Autodesk Fusion 360 part; units mm, degrees
(part 3 of 7)
  line L316 (-32.3491, 29.3042) -> (-32.304, 29.3816)
  spline S628 degree 2 poles (-32.304, 29.3816) (-33.5803, 30.3455) (-33.8371, 31.9456) knots 0 0 0 1 1 1
  spline S629 degree 2 poles (-33.8371, 31.9456) (-33.0539, 30.266) (-32.1923, 29.5954) knots 0 0 0 1 1 1
  line L317 (-32.1923, 29.5954) -> (-32.0902, 29.6502)
  spline S630 degree 2 poles (-32.0902, 29.6502) (-33.142, 30.468) (-33.445, 31.9123) knots 0 0 0 1 1 1
  spline S631 degree 2 poles (-33.445, 31.9123) (-32.5168, 30.1435) (-31.7765, 29.6621) knots 0 0 0 1 1 1
  line L318 (-31.7765, 29.6621) -> (-31.71, 29.7845)
  spline S632 degree 2 poles (-31.71, 29.7845) (-32.8852, 30.77) (-33.0303, 31.7339) knots 0 0 0 1 1 1
  spline S633 degree 2 poles (-33.0303, 31.7339) (-32.3137, 30.4562) (-31.6649, 30.0091) knots 0 0 0 1 1 1
  line L319 (-31.6649, 30.0091) -> (-31.609, 30.0865)
  spline S634 degree 2 poles (-31.609, 30.0865) (-32.2364, 30.6238) (-32.5265, 31.4652) knots 0 0 0 1 1 1
  spline S635 degree 2 poles (-32.5265, 31.4652) (-32.1118, 30.7581) (-31.4403, 30.2326) knots 0 0 0 1 1 1
  line L320 (-31.4403, 30.2326) -> (-31.3844, 30.3337)
  spline S636 degree 2 poles (-31.3844, 30.3337) (-31.8099, 30.871) (-32.1118, 31.4416) knots 0 0 0 1 1 1
  spline S637 degree 2 poles (-32.1118, 31.4416) (-31.5691, 30.7581) (-31.2878, 30.5905) knots 0 0 0 1 1 1
  line L321 (-31.2878, 30.5905) -> (-31.1878, 30.7248)
  spline S638 degree 2 poles (-31.1878, 30.7248) (-31.406, 31.0268) (-31.5284, 31.3868) knots 0 0 0 1 1 1
  spline S639 degree 3 poles (-31.5284, 31.3868) (-31.6519, 31.7446) (-31.0868, 30.9387) (-30.9419, 30.8258) knots 0 0 0 0 1 1 1 1
  line L322 (-30.9419, 30.8258) -> (-30.9074, 30.872)
  spline S640 degree 2 poles (-30.9074, 30.872) (-31.1374, 31.1848) (-31.3049, 31.5093) knots 0 0 0 1 1 1
  spline S641 degree 3 poles (-31.3049, 31.5093) (-31.4725, 31.8327) (-31.2662, 31.6705) (-30.7625, 31.1117) knots 0 0 0 0 1 1 1 1
  line L323 (-30.7625, 31.1117) -> (-30.7066, 31.2234)
  spline S642 degree 2 poles (-30.7066, 31.2234) (-31.2545, 32.2486) (-30.6282, 31.5308) knots 0 0 0 1 1 1
  spline S643 degree 2 poles (-30.6282, 31.5308) (-30.4433, 31.7113) (-30.801, 32.081) knots 0 0 0 1 1 1
  spline S644 degree 3 poles (-30.801, 32.081) (-31.1588, 32.4506) (-30.5207, 32.081) (-30.3198, 31.7349) knots 0 0 0 0 1 1 1 1
  spline S645 degree 3 poles (-30.3198, 31.7349) (-30.1179, 31.3878) (-30.2628, 32.0143) (-30.6454, 32.4377) knots 0 0 0 0 1 1 1 1
  spline S646 degree 3 poles (-30.6454, 32.4377) (-31.0256, 32.8633) (-30.5217, 32.6182) (-30.4541, 32.528) knots 0 0 0 0 1 1 1 1
  spline S647 degree 2 poles (-30.4541, 32.528) (-30.3865, 32.4377) (-30.2199, 32.2368) knots 0 0 0 1 1 1
  spline S648 degree 2 poles (-30.2199, 32.2368) (-30.3231, 32.6859) (-30.6689, 33.0653) knots 0 0 0 1 1 1
  spline S649 degree 3 poles (-30.6689, 33.0653) (-31.017, 33.4457) (-30.5809, 33.1771) (-30.4917, 33.0653) knots 0 0 0 0 1 1 1 1
  spline S650 degree 3 poles (-30.4917, 33.0653) (-30.4015, 32.9535) (-30.2896, 32.874) (-30.1318, 32.6311) knots 0 0 0 0 1 1 1 1
  spline S651 degree 2 poles (-30.1318, 32.6311) (-30.165, 33.0213) (-30.5357, 33.3682) knots 0 0 0 1 1 1
  spline S652 degree 3 poles (-30.5357, 33.3682) (-30.9053, 33.7143) (-30.3574, 33.5467) (-30.0888, 33.1437) knots 0 0 0 0 1 1 1 1
  spline S653 degree 2 poles (-30.0888, 33.1437) (-29.9546, 33.2447) (-30.4917, 33.9497) knots 0 0 0 1 1 1
  spline S654 degree 2 poles (-30.4917, 33.9497) (-31.0289, 34.6546) (-29.9975, 33.58) knots 0 0 0 1 1 1
  spline S655 degree 2 poles (-29.9975, 33.58) (-29.8471, 33.6326) (-30.2887, 34.1303) knots 0 0 0 1 1 1
  spline S656 degree 2 poles (-30.2887, 34.1303) (-30.6474, 34.5331) (-29.9642, 34.04) knots 0 0 0 1 1 1
  spline S657 degree 2 poles (-29.9642, 34.04) (-29.8524, 34.1527) (-30.1102, 34.5203) knots 0 0 0 1 1 1
  spline S658 degree 3 poles (-30.1102, 34.5203) (-30.3563, 34.8727) (-30.0094, 34.6546) (-29.9535, 34.5868) knots 0 0 0 0 1 1 1 1
  spline S659 degree 3 poles (-29.9535, 34.5868) (-29.8954, 34.5203) (-29.8954, 34.9222) (-30.0877, 35.0801) knots 0 0 0 0 1 1 1 1
  spline S660 degree 3 poles (-30.0877, 35.0801) (-30.2779, 35.237) (-30.0094, 35.2478) (-29.9308, 35.1704) knots 0 0 0 0 1 1 1 1
  spline S661 degree 3 poles (-29.9308, 35.1704) (-29.8524, 35.0931) (-29.8524, 35.3048) (-30.0426, 35.5272) knots 0 0 0 0 1 1 1 1
  spline S662 degree 3 poles (-30.0426, 35.5272) (-30.2328, 35.7517) (-29.8858, 35.5842) (-29.8513, 35.5518) knots 0 0 0 0 1 1 1 1
  spline S663 degree 3 poles (-29.8513, 35.5518) (-29.8192, 35.5164) (-29.774, 35.6508) (-29.9083, 35.8206) knots 0 0 0 0 1 1 1 1
  spline S664 degree 3 poles (-29.9083, 35.8206) (-30.0426, 35.9881) (-29.8062, 35.9549) (-29.7611, 35.8754) knots 0 0 0 0 1 1 1 1
  spline S665 degree 3 poles (-29.7611, 35.8754) (-29.717, 35.7959) (-29.6462, 35.9549) (-29.7278, 36.0429) knots 0 0 0 0 1 1 1 1
  spline S666 degree 3 poles (-29.7278, 36.0429) (-29.918, 36.2408) (-29.5345, 36.0623) (-29.4775, 36.158) knots 0 0 0 0 1 1 1 1
  spline S667 degree 3 poles (-29.4775, 36.158) (-29.6622, 36.532) (-29.8342, 36.576) (-30.1265, 36.6222) knots 0 0 0 0 1 1 1 1
  spline S668 degree 3 poles (-30.1265, 36.6222) (-30.4036, 36.6641) (-30.8591, 36.4965) (-31.1136, 36.3847) knots 0 0 0 0 1 1 1 1
  spline S669 degree 2 poles (-31.1136, 36.3847) (-31.161, 36.2397) (-31.0933, 36.0526) knots 0 0 0 1 1 1
  spline S670 degree 3 poles (-31.0933, 36.0526) (-30.9364, 35.6282) (-31.205, 35.9872) (-31.1836, 35.8968) knots 0 0 0 0 1 1 1 1
  spline S671 degree 3 poles (-31.1836, 35.8968) (-31.161, 35.8065) (-31.1266, 35.5509) (-31.2276, 35.683) knots 0 0 0 0 1 1 1 1
  spline S672 degree 2 poles (-31.2276, 35.683) (-31.3285, 35.8195) (-31.4628, 35.9291) knots 0 0 0 1 1 1
  line L324 (-31.4628, 35.9291) -> (-31.4575, 35.9485)
  spline S673 degree 3 poles (-31.4575, 35.9485) (-31.4673, 35.9688) (-31.4706, 35.9917) (-31.4672, 36.014) knots 0 0 0 0 1 1 1 1
  spline S674 degree 3 poles (-31.4672, 36.014) (-31.4274, 36.3073) (-31.4704, 36.4986) (-31.5918, 36.5868) knots 0 0 0 0 1 1 1 1
  spline S675 degree 3 poles (-31.5918, 36.5868) (-31.7142, 36.6749) (-31.9141, 36.6577) (-32.0902, 36.6115) knots 0 0 0 0 1 1 1 1
  spline S676 degree 3 poles (-32.0902, 36.6115) (-32.2696, 36.4061) (-32.4147, 35.6883) (-32.4147, 35.5261) knots 0 0 0 0 1 1 1 1
  spline S677 degree 3 poles (-32.4147, 35.5261) (-32.4147, 35.3606) (-32.2685, 35.0017) (-32.2685, 34.8232) knots 0 0 0 0 1 1 1 1
  spline S678 degree 3 poles (-32.2685, 34.8232) (-32.2685, 34.6449) (-32.3706, 34.6449) (-32.4028, 34.733) knots 0 0 0 0 1 1 1 1
  spline S679 degree 3 poles (-32.4028, 34.733) (-32.4362, 34.8234) (-32.5146, 35.1135) (-32.5941, 35.2478) knots 0 0 0 0 1 1 1 1
  spline S680 degree 3 poles (-32.5941, 35.2478) (-32.6714, 35.3821) (-32.7606, 35.8206) (-32.7606, 35.9634) knots 0 0 0 0 1 1 1 1
  spline S681 degree 3 poles (-32.7606, 35.9634) (-32.7606, 36.1107) (-32.6714, 36.2784) (-32.6714, 36.3793) knots 0 0 0 0 1 1 1 1
  spline S682 degree 3 poles (-32.6714, 36.3793) (-32.6714, 36.4761) (-32.6714, 36.606) (-32.7843, 36.6652) knots 0 0 0 0 1 1 1 1
  spline S683 degree 3 poles (-32.7843, 36.6652) (-32.8667, 36.6822) (-32.952, 36.68) (-33.0335, 36.6588) knots 0 0 0 0 1 1 1 1
  spline S684 degree 3 poles (-33.0335, 36.6588) (-33.0549, 36.6507) (-33.0773, 36.6457) (-33.1001, 36.6436) knots 0 0 0 0 1 1 1 1
  spline S685 degree 3 poles (-33.1001, 36.6436) (-33.0722, 36.5954) (-33.0109, 36.534) (-32.9733, 36.3997) knots 0 0 0 0 1 1 1 1
  spline S686 degree 2 poles (-32.9733, 36.3997) (-32.9175, 36.1977) (-33.0969, 36.2106) knots 0 0 0 1 1 1
  spline S687 degree 2 poles (-33.0969, 36.2106) (-33.0292, 36.0429) (-33.2752, 36.1096) knots 0 0 0 1 1 1
  spline S688 degree 2 poles (-33.2752, 36.1096) (-33.1979, 35.8979) (-33.4772, 36.0323) knots 0 0 0 1 1 1
  spline S689 degree 2 poles (-33.4772, 36.0323) (-33.3998, 35.7195) (-33.7006, 35.9549) knots 0 0 0 1 1 1
  spline S690 degree 2 poles (-33.7006, 35.9549) (-33.4879, 35.4831) (-33.8242, 35.7195) knots 0 0 0 1 1 1
  spline S691 degree 2 poles (-33.8242, 35.7195) (-33.735, 35.3251) (-33.9026, 35.3918) knots 0 0 0 1 1 1
  spline S692 degree 2 poles (-33.9026, 35.3918) (-33.8349, 35.1693) (-34.0251, 35.2263) knots 0 0 0 1 1 1
  spline S693 degree 3 poles (-34.0251, 35.2263) (-34.0025, 35.1576) (-34.0025, 34.9447) (-34.1819, 35.0233) knots 0 0 0 0 1 1 1 1
  spline S694 degree 2 poles (-34.1819, 35.0233) (-34.3613, 35.1027) (-34.3388, 35.2811) knots 0 0 0 1 1 1
  spline S695 degree 3 poles (-34.3388, 35.2811) (-34.1819, 35.2918) (-34.2378, 35.4175) (-34.2496, 35.5604) knots 0 0 0 0 1 1 1 1
  spline S696 degree 3 poles (-34.2496, 35.5604) (-34.2604, 35.7077) (-34.3388, 35.8206) (-34.2937, 35.7851) knots 0 0 0 0 1 1 1 1
  spline S697 degree 3 poles (-34.2937, 35.7851) (-34.1046, 35.6443) (-34.2152, 35.9881) (-34.2937, 36.0763) knots 0 0 0 0 1 1 1 1
  spline S698 degree 3 poles (-34.2937, 36.0763) (-34.3721, 36.1666) (-34.3613, 36.3321) (-34.3162, 36.3009) knots 0 0 0 0 1 1 1 1
  spline S699 degree 3 poles (-34.3162, 36.3009) (-34.0874, 36.129) (-34.1819, 36.3665) (-34.2937, 36.6007) knots 0 0 0 0 1 1 1 1
  spline S700 degree 2 poles (-34.2937, 36.6007) (-34.4065, 36.8382) (-34.1927, 36.7244) knots 0 0 0 1 1 1
  spline S701 degree 2 poles (-34.1927, 36.7244) (-34.0702, 36.5791) (-34.1712, 36.8146) knots 0 0 0 1 1 1
  spline S702 degree 3 poles (-34.1712, 36.8146) (-34.2851, 37.079) (-34.1336, 37.079) (-34.0852, 37.0746) knots 0 0 0 0 1 1 1 1
  spline S703 degree 3 poles (-34.0852, 37.0746) (-34.0928, 37.2304) (-34.1346, 37.4508) (-34.3022, 37.4948) knots 0 0 0 0 1 1 1 1
  spline S704 degree 3 poles (-34.3022, 37.4948) (-34.5203, 37.5571) (-35.166, 37.2067) (-35.5925, 36.9779) knots 0 0 0 0 1 1 1 1
  spline S705 degree 2 poles (-31.3082, 35.3262) (-31.2631, 35.5948) (-31.4425, 35.7861) knots 0 0 0 1 1 1
  spline S706 degree 3 poles (-31.4425, 35.7861) (-31.6219, 35.9773) (-31.5768, 35.7968) (-31.5435, 35.7088) knots 0 0 0 0 1 1 1 1
  spline S707 degree 3 poles (-31.5435, 35.7088) (-31.509, 35.6174) (-31.4425, 35.4389) (-31.3082, 35.3262) knots 0 0 0 0 1 1 1 1
  spline S708 degree 2 poles (-31.5317, 35.1919) (-31.5101, 35.5378) (-31.7003, 35.5067) knots 0 0 0 1 1 1
  spline S709 degree 3 poles (-31.7003, 35.5067) (-31.767, 35.4959) (-31.6327, 35.3047) (-31.5317, 35.1919) knots 0 0 0 0 1 1 1 1
  spline S710 degree 2 poles (-31.6433, 34.9016) (-31.6433, 35.1488) (-31.7776, 35.2144) knots 0 0 0 1 1 1
  spline S711 degree 3 poles (-31.7776, 35.2144) (-32.043, 35.3467) (-31.7111, 34.9586) (-31.6433, 34.9016) knots 0 0 0 0 1 1 1 1
  spline S712 degree 2 poles (-31.7776, 34.7104) (-31.8121, 34.9899) (-31.9345, 34.9458) knots 0 0 0 1 1 1
  spline S713 degree 3 poles (-31.9345, 34.9458) (-32.058, 34.9016) (-31.8335, 34.7341) (-31.7776, 34.7104) knots 0 0 0 0 1 1 1 1
  spline S714 degree 2 poles (-31.9689, 36.4191) (-31.7787, 36.4319) (-31.6884, 36.3857) knots 0 0 0 1 1 1
  spline S715 degree 2 poles (-31.6884, 36.3857) (-31.7454, 36.577) (-31.9689, 36.4191) knots 0 0 0 1 1 1
  spline S716 degree 2 poles (-31.7111, 36.2664) (-31.8572, 36.3922) (-31.9689, 36.3126) knots 0 0 0 1 1 1
  spline S717 degree 2 poles (-31.9689, 36.3126) (-32.0807, 36.2331) (-31.7111, 36.2664) knots 0 0 0 1 1 1
  spline S718 degree 2 poles (-31.7562, 36.1547) (-31.8572, 36.1107) (-31.9345, 36.1107) knots 0 0 0 1 1 1
  spline S719 degree 3 poles (-31.9345, 36.1107) (-32.0129, 36.1107) (-31.8678, 35.9978) (-31.7562, 36.1547) knots 0 0 0 0 1 1 1 1
  spline S720 degree 2 poles (-34.2292, 34.9791) (-34.3635, 34.9685) (-34.3635, 34.8781) knots 0 0 0 1 1 1
  spline S721 degree 2 poles (-34.3635, 34.8781) (-34.2958, 34.935) (-34.1948, 34.8448) knots 0 0 0 1 1 1
  spline S722 degree 2 poles (-34.1948, 34.8448) (-34.0949, 34.7545) (-34.2292, 34.9791) knots 0 0 0 1 1 1
  spline S723 degree 2 poles (-31.5209, 31.9004) (-31.6424, 32.0477) (-31.6552, 32.1272) knots 0 0 0 1 1 1
  spline S724 degree 3 poles (-31.6552, 32.1272) (-31.6659, 32.2035) (-31.5209, 32.0939) (-31.5209, 31.9004) knots 0 0 0 0 1 1 1 1
  spline S725 degree 2 poles (-31.6499, 31.4523) (-31.7723, 31.5985) (-31.7841, 31.6759) knots 0 0 0 1 1 1
  spline S726 degree 3 poles (-31.7841, 31.6759) (-31.7949, 31.7543) (-31.6499, 31.6447) (-31.6499, 31.4523) knots 0 0 0 0 1 1 1 1
  spline S727 degree 2 poles (-31.0676, 31.9445) (-31.1911, 32.0917) (-31.2019, 32.1691) knots 0 0 0 1 1 1
  spline S728 degree 3 poles (-31.2019, 32.1691) (-31.2147, 32.2475) (-31.0676, 32.1379) (-31.0676, 31.9445) knots 0 0 0 0 1 1 1 1
  spline S729 degree 2 poles (-31.0117, 32.3496) (-31.1352, 32.4968) (-31.146, 32.5721) knots 0 0 0 1 1 1
  spline S730 degree 3 poles (-31.146, 32.5721) (-31.1578, 32.6515) (-31.0117, 32.5409) (-31.0117, 32.3496) knots 0 0 0 0 1 1 1 1
  spline S731 degree 2 poles (-30.8946, 32.7655) (-30.9505, 32.8536) (-30.9945, 32.8998) knots 0 0 0 1 1 1
  spline S732 degree 3 poles (-30.9945, 32.8998) (-31.0396, 32.9438) (-30.827, 32.9438) (-30.8946, 32.7655) knots 0 0 0 0 1 1 1 1
  spline S733 degree 2 poles (-31.3641, 32.283) (-31.4209, 32.3711) (-31.465, 32.4173) knots 0 0 0 1 1 1
  spline S734 degree 3 poles (-31.465, 32.4173) (-31.5092, 32.4614) (-31.2963, 32.4614) (-31.3641, 32.283) knots 0 0 0 0 1 1 1 1
  spline S735 degree 2 poles (-32.2031, 31.6995) (-32.2601, 31.7919) (-32.3041, 31.8338) knots 0 0 0 1 1 1
  spline S736 degree 3 poles (-32.3041, 31.8338) (-32.3493, 31.88) (-32.1364, 31.88) (-32.2031, 31.6995) knots 0 0 0 0 1 1 1 1
  spline S737 degree 2 poles (-32.606, 31.6909) (-32.663, 31.779) (-32.707, 31.8252) knots 0 0 0 1 1 1
  spline S738 degree 3 poles (-32.707, 31.8252) (-32.7521, 31.8693) (-32.5383, 31.8693) (-32.606, 31.6909) knots 0 0 0 0 1 1 1 1
  spline S739 degree 2 poles (-30.4014, 34.3977) (-30.4574, 34.486) (-30.5025, 34.5322) knots 0 0 0 1 1 1
  spline S740 degree 3 poles (-30.5025, 34.5322) (-30.5476, 34.5762) (-30.3349, 34.5762) (-30.4014, 34.3977) knots 0 0 0 0 1 1 1 1
  spline S741 degree 2 poles (-30.2458, 34.7803) (-30.3006, 34.8685) (-30.3466, 34.9147) knots 0 0 0 1 1 1
  spline S742 degree 3 poles (-30.3466, 34.9147) (-30.3897, 34.9588) (-30.178, 34.9588) (-30.2458, 34.7803) knots 0 0 0 0 1 1 1 1
  line L325 (-32.4609, 32.182) -> (-32.405, 32.1379)
  line L326 (-32.405, 32.1379) -> (-32.3944, 32.2615)
  line L327 (-32.3944, 32.2615) -> (-32.4609, 32.2723)
  line L328 (-32.4609, 32.2723) -> (-32.4609, 32.182)
  line L329 (-31.8368, 32.3625) -> (-31.7809, 32.3163)
  line L330 (-31.7809, 32.3163) -> (-31.769, 32.4399)
  line L331 (-31.769, 32.4399) -> (-31.8368, 32.4528)
  line L332 (-31.8368, 32.4528) -> (-31.8368, 32.3625)
  line L333 (-30.972, 34.0163) -> (-30.9172, 33.9744)
  line L334 (-30.9172, 33.9744) -> (-30.9053, 34.0959)
  line L335 (-30.9053, 34.0959) -> (-30.972, 34.1087)
  line L336 (-30.972, 34.1087) -> (-30.972, 34.0163)
  line L337 (-30.7152, 33.7605) -> (-30.6583, 33.7144)
  line L338 (-30.6583, 33.7144) -> (-30.6486, 33.8401)
  line L339 (-30.6486, 33.8401) -> (-30.7152, 33.8487)
  line L340 (-30.7152, 33.8487) -> (-30.7152, 33.7605)
  spline S743 degree 3 poles (-43.5424, 38.6843) (-43.5791, 38.6514) (-43.6163, 38.6192) (-43.6541, 38.5875) knots 0 0 0 0 1 1 1 1
  line L341 (-43.6541, 38.5875) -> (-43.6541, 33.162)
  spline S744 degree 3 poles (-43.6541, 33.162) (-43.6187, 33.25) (-43.5811, 33.3381) (-43.5424, 33.4285) knots 0 0 0 0 1 1 1 1
  line L342 (-43.5424, 33.4285) -> (-43.5424, 38.6843)
  line L343 (-44.4846, 37.8107) -> (-44.5974, 37.6956)
  line L344 (-44.5974, 37.6956) -> (-44.5974, 32.4302)
  line L345 (-44.5974, 32.4302) -> (-44.4846, 32.4011)
  line L346 (-44.4846, 32.4011) -> (-44.4846, 37.8107)
  line L347 (-43.2276, 38.9401) -> (-43.3404, 38.8477)
  line L348 (-43.3404, 38.8477) -> (-43.3404, 33.84)
  spline S745 degree 3 poles (-43.3404, 33.84) (-43.3039, 33.9067) (-43.2663, 33.9764) (-43.2276, 34.0431) knots 0 0 0 0 1 1 1 1
  line L349 (-43.2276, 34.0431) -> (-43.2276, 38.9401)
  spline S746 degree 3 poles (-44.1698, 38.1213) (-44.2084, 38.0858) (-44.246, 38.0493) (-44.2826, 38.0117) knots 0 0 0 0 1 1 1 1
  line L350 (-44.2826, 38.0117) -> (-44.2826, 32.341)
  line L351 (-44.2826, 32.341) -> (-44.1698, 32.3076)
  line L352 (-44.1698, 32.3076) -> (-44.1698, 38.1213)
  spline S747 degree 3 poles (-45.4267, 36.7317) (-45.4654, 36.6813) (-45.503, 36.6329) (-45.5395, 36.5824) knots 0 0 0 0 1 1 1 1
  line L353 (-45.5395, 36.5824) -> (-45.5395, 32.6999)
  line L354 (-45.5395, 32.6999) -> (-45.4267, 32.6687)
  line L355 (-45.4267, 32.6687) -> (-45.4267, 36.7317)
  spline S748 degree 3 poles (-45.7404, 36.3062) (-45.7785, 36.2522) (-45.8161, 36.1977) (-45.8532, 36.1429) knots 0 0 0 0 1 1 1 1
  line L356 (-45.8532, 36.1429) -> (-45.8532, 32.7913)
  line L357 (-45.8532, 32.7913) -> (-45.7404, 32.76)
  line L358 (-45.7404, 32.76) -> (-45.7404, 36.3062)
  spline S749 degree 3 poles (-45.1119, 37.1208) (-45.1507, 37.0762) (-45.1883, 37.0307) (-45.2247, 36.9843) knots 0 0 0 0 1 1 1 1
  line L359 (-45.2247, 36.9843) -> (-45.2247, 32.6107)
  line L360 (-45.2247, 32.6107) -> (-45.1119, 32.5795)
  line L361 (-45.1119, 32.5795) -> (-45.1119, 37.1208)
  line L362 (-44.7993, 37.4797) -> (-44.9111, 37.3529)
  line L363 (-44.9111, 37.3529) -> (-44.9111, 32.5193)
  line L364 (-44.9111, 32.5193) -> (-44.7993, 32.4882)
  line L365 (-44.7993, 32.4882) -> (-44.7993, 37.4797)
  spline S750 degree 3 poles (-40.7137, 40.525) (-40.7518, 40.5077) (-40.7894, 40.4894) (-40.8265, 40.4702) knots 0 0 0 0 1 1 1 1
  line L366 (-40.8265, 40.4702) -> (-40.8265, 36.9381)
  line L367 (-40.8265, 36.9381) -> (-40.7137, 37.0198)
  line L368 (-40.7137, 37.0198) -> (-40.7137, 40.525)
  line L369 (-41.6559, 40.0146) -> (-41.7687, 39.9481)
  line L370 (-41.7687, 39.9481) -> (-41.7687, 36.057)
  line L371 (-41.7687, 36.057) -> (-41.6559, 36.1869)
  line L372 (-41.6559, 36.1869) -> (-41.6559, 40.0146)
  line L373 (-40.0853, 40.8206) -> (-40.1981, 40.77)
  line L374 (-40.1981, 40.77) -> (-40.1981, 37.3324)
  spline S751 degree 3 poles (-40.1981, 37.3324) (-40.1594, 37.3518) (-40.1218, 37.3722) (-40.0853, 37.3894) knots 0 0 0 0 1 1 1 1
  line L375 (-40.0853, 37.3894) -> (-40.0853, 40.8206)
  line L376 (-40.399, 40.6776) -> (-40.5118, 40.6229)
  line L377 (-40.5118, 40.6229) -> (-40.5118, 37.1497)
  spline S752 degree 3 poles (-40.5118, 37.1497) (-40.4742, 37.1724) (-40.4366, 37.1981) (-40.399, 37.2186) knots 0 0 0 0 1 1 1 1
  line L378 (-40.399, 37.2186) -> (-40.399, 40.6776)
  spline S753 degree 3 poles (-42.5991, 39.4064) (-42.6376, 39.3816) (-42.6748, 39.355) (-42.7109, 39.3269) knots 0 0 0 0 1 1 1 1
  line L379 (-42.7109, 39.3269) -> (-42.7109, 34.849)
  line L380 (-42.7109, 34.849) -> (-42.5991, 35.0059)
  line L381 (-42.5991, 35.0059) -> (-42.5991, 39.4064)
  spline S754 degree 3 poles (-42.9128, 39.1797) (-42.9509, 39.1525) (-42.9886, 39.1245) (-43.0256, 39.0958) knots 0 0 0 0 1 1 1 1
  line L382 (-43.0256, 39.0958) -> (-43.0256, 34.3817)
  line L383 (-43.0256, 34.3817) -> (-42.9128, 34.5558)
  line L384 (-42.9128, 34.5558) -> (-42.9128, 39.1797)
  line L385 (-41.9707, 39.8233) -> (-42.0835, 39.7524)
  line L386 (-42.0835, 39.7524) -> (-42.0835, 35.6764)
  line L387 (-42.0835, 35.6764) -> (-41.9707, 35.8151)
  line L388 (-41.9707, 35.8151) -> (-41.9707, 39.8233)
  spline S755 degree 3 poles (-42.2844, 39.6223) (-42.3225, 39.5973) (-42.3601, 39.5716) (-42.3972, 39.545) knots 0 0 0 0 1 1 1 1
  line L389 (-42.3972, 39.545) -> (-42.3972, 35.2778)
  line L390 (-42.3972, 35.2778) -> (-42.2844, 35.4229)
  line L391 (-42.2844, 35.4229) -> (-42.2844, 39.6223)
  line L392 (-41.0274, 40.365) -> (-41.1402, 40.3038)
  line L393 (-41.1402, 40.3038) -> (-41.1402, 36.6899)
  spline S756 degree 3 poles (-41.1402, 36.6899) (-41.1026, 36.7211) (-41.065, 36.7532) (-41.0274, 36.7823) knots 0 0 0 0 1 1 1 1
  line L394 (-41.0274, 36.7823) -> (-41.0274, 40.365)
  spline S757 degree 3 poles (-29.4024, 41.7502) (-29.44, 41.7608) (-29.4775, 41.7694) (-29.5151, 41.777) knots 0 0 0 0 1 1 1 1
  line L395 (-29.5151, 41.777) -> (-29.5151, 36.6179)
  spline S758 degree 3 poles (-29.5151, 36.6179) (-29.473, 36.5795) (-29.4352, 36.5365) (-29.4024, 36.49) knots 0 0 0 0 1 1 1 1
  line L396 (-29.4024, 36.49) -> (-29.4024, 41.7502)
  spline S759 degree 3 poles (-30.0309, 41.8866) (-30.0684, 41.8952) (-30.106, 41.9016) (-30.1436, 41.908) knots 0 0 0 0 1 1 1 1
  line L397 (-30.1436, 41.908) -> (-30.1436, 36.8607)
  line L398 (-30.1436, 36.8607) -> (-30.0932, 36.8543)
  line L399 (-30.0932, 36.8543) -> (-30.0298, 36.8435)
  line L400 (-30.0298, 36.8435) -> (-30.0298, 41.8866)
  line L401 (-30.0298, 41.8866) -> (-30.0309, 41.8866)
  spline S760 degree 3 poles (-29.0887, 41.6727) (-29.1263, 41.6835) (-29.1627, 41.6921) (-29.2003, 41.6996) knots 0 0 0 0 1 1 1 1
  line L402 (-29.2003, 41.6996) -> (-29.2003, 36.1171)
  spline S761 degree 3 poles (-29.2003, 36.1171) (-29.1616, 36.0242) (-29.1254, 35.9303) (-29.0918, 35.8356) knots 0 0 0 0 1 1 1 1
  line L403 (-29.0918, 35.8356) -> (-29.0876, 35.8206)
  line L404 (-29.0876, 35.8206) -> (-29.0887, 41.6727)
  line L405 (-33.8006, 42.2036) -> (-33.9144, 42.1993)
  line L406 (-33.9144, 42.1993) -> (-33.9144, 37.4033)
  spline S762 degree 3 poles (-33.9144, 37.4033) (-33.8667, 37.2679) (-33.8449, 37.1246) (-33.85, 36.9811) knots 0 0 0 0 1 1 1 1
  line L407 (-33.85, 36.9811) -> (-33.8006, 36.9639)
  line L408 (-33.8006, 36.9639) -> (-33.8006, 42.2036)
  line L409 (-35.7988, 42.0381) -> (-35.7988, 37.1336)
  line L410 (-35.7988, 37.1336) -> (-35.7042, 37.1842)
  line L411 (-35.7042, 37.1842) -> (-35.686, 37.1948)
  line L412 (-35.686, 37.1948) -> (-35.686, 42.0531)
  line L413 (-35.686, 42.0531) -> (-35.7988, 42.0381)
  spline S763 degree 3 poles (-46.0552, 35.8356) (-46.0936, 35.7751) (-46.1312, 35.7142) (-46.168, 35.6529) knots 0 0 0 0 1 1 1 1
  line L414 (-46.168, 35.6529) -> (-46.168, 32.8804)
  line L415 (-46.168, 32.8804) -> (-46.0552, 32.847)
  line L416 (-46.0552, 32.847) -> (-46.0552, 35.8356)
  line L417 (-27.9435, 38.2577) -> (-27.9435, 35.2756)
  spline S764 degree 3 poles (-27.9435, 35.2756) (-27.9274, 35.2775) (-27.9112, 35.2781) (-27.8951, 35.2778) knots 0 0 0 0 1 1 1 1
  spline S765 degree 3 poles (-27.8951, 35.2778) (-27.8746, 35.2778) (-27.8553, 35.28) (-27.8306, 35.2864) knots 0 0 0 0 1 1 1 1
  line L418 (-27.8306, 35.2864) -> (-27.8306, 38.1706)
  spline S766 degree 3 poles (-27.8306, 38.1706) (-27.8715, 38.1953) (-27.9093, 38.2245) (-27.9435, 38.2577) knots 0 0 0 0 1 1 1 1
  spline S767 degree 3 poles (-28.1809, 38.8186) (-28.1809, 38.9197) (-28.167, 39.0055) (-28.1443, 39.0786) knots 0 0 0 0 1 1 1 1
  line L419 (-28.1443, 39.0786) -> (-28.1443, 41.3976)
  line L420 (-28.1443, 41.3976) -> (-28.2581, 41.433)
  line L421 (-28.2581, 41.433) -> (-28.2581, 35.2692)
  spline S768 degree 3 poles (-28.2581, 35.2692) (-28.2196, 35.267) (-28.1819, 35.2692) (-28.1443, 35.2692) knots 0 0 0 0 1 1 1 1
  line L422 (-28.1443, 35.2692) -> (-28.1443, 38.5789)
  spline S769 degree 3 poles (-28.1443, 38.5789) (-28.1687, 38.6565) (-28.181, 38.7373) (-28.1809, 38.8186) knots 0 0 0 0 1 1 1 1
  line L423 (-27.315, 37.5613) -> (-27.315, 35.5927)
  spline S770 degree 3 poles (-27.315, 35.5927) (-27.2989, 35.606) (-27.2842, 35.6207) (-27.271, 35.6368) knots 0 0 0 0 1 1 1 1
  spline S771 degree 3 poles (-27.271, 35.6368) (-27.2483, 35.6561) (-27.2269, 35.6808) (-27.2032, 35.7077) knots 0 0 0 0 1 1 1 1
  line L424 (-27.2032, 35.7077) -> (-27.2032, 37.4055)
  line L425 (-27.2032, 37.4055) -> (-27.315, 37.5613)
  line L426 (-46.6837, 34.7029) -> (-46.7965, 34.4611)
  line L427 (-46.7965, 34.4611) -> (-46.7965, 33.0673)
  line L428 (-46.7965, 33.0673) -> (-46.718, 33.046)
  spline S772 degree 3 poles (-46.718, 33.046) (-46.7148, 33.0438) (-46.7116, 33.0416) (-46.7084, 33.0416) knots 0 0 0 0 1 1 1 1
  line L429 (-46.7084, 33.0416) -> (-46.6837, 33.033)
  line L430 (-46.6837, 33.033) -> (-46.6837, 34.7029)
  spline S773 degree 3 poles (-27.9435, 39.3978) (-27.9093, 39.4273) (-27.8718, 39.4526) (-27.8317, 39.4731) knots 0 0 0 0 1 1 1 1
  line L431 (-27.8317, 39.4731) -> (-27.8317, 41.2923)
  spline S774 degree 3 poles (-27.8317, 41.2923) (-27.8682, 41.3052) (-27.9059, 41.3192) (-27.9435, 41.33) knots 0 0 0 0 1 1 1 1
  line L432 (-27.9435, 41.33) -> (-27.9435, 39.3978)
  line L433 (-46.3689, 35.309) -> (-46.4817, 35.1037)
  line L434 (-46.4817, 35.1037) -> (-46.4817, 32.9738)
  line L435 (-46.4817, 32.9738) -> (-46.3689, 32.9427)
  line L436 (-46.3689, 32.9427) -> (-46.3689, 35.309)
  line L437 (-41.455, 40.1297) -> (-41.455, 36.3997)
  line L438 (-41.455, 36.3997) -> (-41.3422, 36.5093)
  line L439 (-41.3422, 36.5093) -> (-41.3422, 40.1952)
  spline S775 degree 3 poles (-41.3422, 40.1952) (-41.3798, 40.1737) (-41.4174, 40.1532) (-41.455, 40.1297) knots 0 0 0 0 1 1 1 1
  spline S776 degree 3 poles (-36.9429, 41.8318) (-36.9805, 41.8253) (-37.0181, 41.8167) (-37.0546, 41.8092) knots 0 0 0 0 1 1 1 1
  line L440 (-37.0546, 41.8092) -> (-37.0546, 37.1325)
  spline S777 degree 3 poles (-37.0546, 37.1325) (-37.0504, 37.1283) (-37.045, 37.1239) (-37.0407, 37.1175) knots 0 0 0 0 1 1 1 1
  spline S778 degree 3 poles (-37.0407, 37.1175) (-37.0262, 37.1021) (-37.0162, 37.083) (-37.0119, 37.0624) knots 0 0 0 0 1 1 1 1
  spline S779 degree 3 poles (-37.0119, 37.0624) (-37.0075, 37.0418) (-37.0089, 37.0203) (-37.016, 37.0004) knots 0 0 0 0 1 1 1 1
  spline S780 degree 3 poles (-37.016, 37.0004) (-37.0342, 36.9478) (-37.0482, 36.8554) (-37.0203, 36.8156) knots 0 0 0 0 1 1 1 1
  spline S781 degree 3 poles (-37.0203, 36.8156) (-37.0052, 36.7962) (-36.9719, 36.7909) (-36.9418, 36.7887) knots 0 0 0 0 1 1 1 1
  line L441 (-36.9418, 36.7887) -> (-36.9429, 41.8318)
  line L442 (-36.742, 41.8748) -> (-36.742, 36.7812)
  line L443 (-36.742, 36.7812) -> (-36.7367, 36.7812)
  spline S782 degree 3 poles (-36.7367, 36.7812) (-36.6948, 36.779) (-36.6625, 36.7768) (-36.6292, 36.779) knots 0 0 0 0 1 1 1 1
  line L444 (-36.6292, 36.779) -> (-36.6292, 41.8984)
  spline S783 degree 3 poles (-36.6292, 41.8984) (-36.6668, 41.8887) (-36.7044, 41.8823) (-36.742, 41.8748) knots 0 0 0 0 1 1 1 1
  line L445 (-43.9689, 38.3082) -> (-43.9689, 32.2507)
  line L446 (-43.9689, 32.2507) -> (-43.9356, 32.2399)
  spline S784 degree 3 poles (-43.9356, 32.2399) (-43.912, 32.3495) (-43.8851, 32.4559) (-43.855, 32.5613) knots 0 0 0 0 1 1 1 1
  line L447 (-43.855, 32.5613) -> (-43.855, 38.4125)
  spline S785 degree 3 poles (-43.855, 38.4125) (-43.8935, 38.3783) (-43.9314, 38.3435) (-43.9689, 38.3082) knots 0 0 0 0 1 1 1 1
  spline S786 degree 3 poles (-32.23, 42.1746) (-32.2665, 42.1768) (-32.3041, 42.1768) (-32.3416, 42.181) knots 0 0 0 0 1 1 1 1
  line L448 (-32.3416, 42.181) -> (-32.3416, 36.7812)
  spline S787 degree 3 poles (-32.3416, 36.7812) (-32.3083, 36.7962) (-32.2696, 36.8081) (-32.23, 36.821) knots 0 0 0 0 1 1 1 1
  line L449 (-32.23, 36.821) -> (-32.23, 42.1746)
  line L450 (-31.2878, 42.0865) -> (-31.3996, 42.0993)
  line L451 (-31.3996, 42.0993) -> (-31.3996, 36.7297)
  spline S788 degree 3 poles (-31.3996, 36.7297) (-31.3519, 36.6838) (-31.314, 36.629) (-31.2878, 36.5684) knots 0 0 0 0 1 1 1 1
  line L452 (-31.2878, 36.5684) -> (-31.2878, 42.0865)
  line L453 (-31.6004, 42.1198) -> (-31.7133, 42.1327)
  line L454 (-31.7133, 42.1327) -> (-31.7133, 36.8768)
  spline S789 degree 3 poles (-31.7133, 36.8768) (-31.675, 36.8704) (-31.6374, 36.8615) (-31.6004, 36.8499) knots 0 0 0 0 1 1 1 1
  line L455 (-31.6004, 36.8499) -> (-31.6004, 42.1198)
  line L456 (-30.9719, 42.0445) -> (-31.0848, 42.0617)
  line L457 (-31.0848, 42.0617) -> (-31.0848, 36.6533)
  spline S790 degree 3 poles (-31.0848, 36.6533) (-31.0504, 36.6683) (-31.0117, 36.6824) (-30.9719, 36.6973) knots 0 0 0 0 1 1 1 1
  line L458 (-30.9719, 36.6973) -> (-30.9719, 42.0445)
  line L459 (-30.6582, 42.0005) -> (-30.7711, 42.0155)
  line L460 (-30.7711, 42.0155) -> (-30.7711, 36.7662)
  line L461 (-30.7711, 36.7662) -> (-30.6582, 36.7973)
  line L462 (-30.6582, 36.7973) -> (-30.6582, 42.0005)
  spline S791 degree 3 poles (-31.9152, 42.1488) (-31.9517, 42.153) (-31.9904, 42.1552) (-32.0279, 42.1574) knots 0 0 0 0 1 1 1 1
  line L463 (-32.0279, 42.1574) -> (-32.0279, 36.8682)
  spline S792 degree 3 poles (-32.0279, 36.8682) (-31.9904, 36.8725) (-31.9528, 36.8789) (-31.9152, 36.8811) knots 0 0 0 0 1 1 1 1
  line L464 (-31.9152, 36.8811) -> (-31.9152, 42.1488)
  line L465 (-32.5437, 42.1885) -> (-32.6564, 42.195)
  line L466 (-32.6564, 42.195) -> (-32.6564, 36.8725)
  spline S793 degree 3 poles (-32.6564, 36.8725) (-32.6169, 36.8596) (-32.5789, 36.8419) (-32.5437, 36.8199) knots 0 0 0 0 1 1 1 1
  line L467 (-32.5437, 36.8199) -> (-32.5437, 42.1885)
  spline S794 degree 3 poles (-33.1721, 42.2078) (-33.2108, 42.21) (-33.2473, 42.21) (-33.286, 42.21) knots 0 0 0 0 1 1 1 1
  line L468 (-33.286, 42.21) -> (-33.286, 36.864)
  spline S795 degree 3 poles (-33.286, 36.864) (-33.2473, 36.864) (-33.2108, 36.8661) (-33.1732, 36.8704) knots 0 0 0 0 1 1 1 1
  line L469 (-33.1732, 36.8704) -> (-33.1721, 42.2078)
  line L470 (-32.8574, 36.9102) -> (-32.8574, 42.2014)
  spline S796 degree 3 poles (-32.8574, 42.2014) (-32.895, 42.2014) (-32.9325, 42.2036) (-32.9701, 42.2057) knots 0 0 0 0 1 1 1 1
  line L471 (-32.9701, 42.2057) -> (-32.9701, 36.9058)
  spline S797 degree 3 poles (-32.9701, 36.9058) (-32.9315, 36.9102) (-32.8939, 36.9122) (-32.8574, 36.9102) knots 0 0 0 0 1 1 1 1
  line L472 (-28.7739, 41.5889) -> (-28.8866, 41.6179)
  line L473 (-28.8866, 41.6179) -> (-28.8866, 35.4895)
  spline S798 degree 3 poles (-28.8866, 35.4895) (-28.8526, 35.4552) (-28.8148, 35.4249) (-28.7739, 35.3993) knots 0 0 0 0 1 1 1 1
  line L474 (-28.7739, 35.3993) -> (-28.7739, 41.5889)
  spline S799 degree 3 poles (-26.8884, 36.967) (-26.924, 37.0176) (-26.9615, 37.0724) (-27.0013, 37.1239) knots 0 0 0 0 1 1 1 1
  line L475 (-27.0013, 37.1239) -> (-27.0013, 35.9967)
  spline S800 degree 3 poles (-27.0013, 35.9967) (-26.9509, 36.0935) (-26.91, 36.202) (-26.8884, 36.3202) knots 0 0 0 0 1 1 1 1
  line L476 (-26.8884, 36.3202) -> (-26.8884, 36.967)
  line L477 (-27.5169, 37.8365) -> (-27.6298, 37.9857)
  line L478 (-27.6298, 37.9857) -> (-27.6298, 35.3659)
  spline S801 degree 3 poles (-27.6298, 35.3659) (-27.5933, 35.3852) (-27.5556, 35.4079) (-27.5169, 35.4325) knots 0 0 0 0 1 1 1 1
  line L479 (-27.5169, 35.4325) -> (-27.5169, 37.8365)
  spline S802 degree 3 poles (-30.3445, 41.9457) (-30.3832, 41.9543) (-30.4197, 41.9586) (-30.4573, 41.965) knots 0 0 0 0 1 1 1 1
  line L480 (-30.4573, 41.965) -> (-30.4573, 36.8413)
  spline S803 degree 3 poles (-30.4573, 36.8413) (-30.4197, 36.8479) (-30.3821, 36.8521) (-30.3445, 36.8565) knots 0 0 0 0 1 1 1 1
  line L481 (-30.3445, 36.8565) -> (-30.3445, 41.9457)
  spline S804 degree 3 poles (-46.9973, 33.9808) (-47.0963, 33.7274) (-47.1859, 33.4704) (-47.2659, 33.2102) knots 0 0 0 0 1 1 1 1
  line L482 (-47.2659, 33.2102) -> (-46.9973, 33.1307)
  line L483 (-46.9973, 33.1307) -> (-46.9973, 33.9808)
  spline S805 degree 3 poles (-29.7172, 41.8222) (-29.7547, 41.8307) (-29.7912, 41.8393) (-29.8288, 41.8446) knots 0 0 0 0 1 1 1 1
  line L484 (-29.8288, 41.8446) -> (-29.8288, 36.7973)
  spline S806 degree 3 poles (-29.8288, 36.7973) (-29.7901, 36.7823) (-29.7526, 36.7704) (-29.7172, 36.7532) knots 0 0 0 0 1 1 1 1
  line L485 (-29.7172, 36.7532) -> (-29.7172, 41.8222)
  spline S807 degree 3 poles (-28.4591, 41.4964) (-28.4967, 41.5094) (-28.5344, 41.5191) (-28.5729, 41.5299) knots 0 0 0 0 1 1 1 1
  line L486 (-28.5729, 41.5299) -> (-28.5729, 35.309)
  spline S808 degree 3 poles (-28.5729, 35.309) (-28.5359, 35.2978) (-28.4977, 35.2901) (-28.4591, 35.2864) knots 0 0 0 0 1 1 1 1
  line L487 (-28.4591, 35.2864) -> (-28.4591, 41.4964)
  spline S809 degree 3 poles (-33.4869, 42.21) (-33.5245, 42.2078) (-33.561, 42.2078) (-33.5986, 42.2078) knots 0 0 0 0 1 1 1 1
  line L488 (-33.5986, 42.2078) -> (-33.5986, 36.9036)
  spline S810 degree 3 poles (-33.5986, 36.9036) (-33.5621, 36.895) (-33.5245, 36.8886) (-33.4869, 36.8811) knots 0 0 0 0 1 1 1 1
  line L489 (-33.4869, 36.8811) -> (-33.4869, 42.21)
  spline S811 degree 3 poles (-36.3145, 41.9565) (-36.3521, 41.95) (-36.3897, 41.9435) (-36.4273, 41.9349) knots 0 0 0 0 1 1 1 1
  line L490 (-36.4273, 41.9349) -> (-36.4273, 36.8327)
  spline S812 degree 3 poles (-36.4273, 36.8327) (-36.3939, 36.8457) (-36.3585, 36.8596) (-36.3145, 36.879) knots 0 0 0 0 1 1 1 1
  line L491 (-36.3145, 36.879) -> (-36.3145, 41.9565)
  spline S813 degree 3 poles (-37.5714, 41.6857) (-37.609, 41.6771) (-37.6466, 41.6685) (-37.6842, 41.6566) knots 0 0 0 0 1 1 1 1
  line L492 (-37.6842, 41.6566) -> (-37.6842, 36.9844)
  spline S814 degree 3 poles (-37.6842, 36.9844) (-37.6456, 36.9981) (-37.6079, 37.0142) (-37.5714, 37.0326) knots 0 0 0 0 1 1 1 1
  line L493 (-37.5714, 37.0326) -> (-37.5714, 41.6857)
  spline S815 degree 3 poles (-38.1999, 41.5138) (-38.2378, 41.5028) (-38.2754, 41.491) (-38.3127, 41.4782) knots 0 0 0 0 1 1 1 1
  line L494 (-38.3127, 41.4782) -> (-38.3127, 37.6945)
  spline S816 degree 3 poles (-38.3127, 37.6945) (-38.2716, 37.6708) (-38.2337, 37.6419) (-38.1999, 37.6086) knots 0 0 0 0 1 1 1 1
  line L495 (-38.1999, 37.6086) -> (-38.1999, 41.5138)
  line L496 (-37.8862, 41.604) -> (-37.9979, 41.5728)
  line L497 (-37.9979, 41.5728) -> (-37.9979, 36.9113)
  spline S817 degree 3 poles (-37.9979, 36.9113) (-37.9603, 36.9131) (-37.9229, 36.9181) (-37.8862, 36.9263) knots 0 0 0 0 1 1 1 1
  line L498 (-37.8862, 36.9263) -> (-37.8862, 41.604)
  line L499 (-38.5146, 41.417) -> (-38.6264, 41.3793)
  line L500 (-38.6264, 41.3793) -> (-38.6264, 37.788)
  spline S818 degree 3 poles (-38.6264, 37.788) (-38.5888, 37.784) (-38.5514, 37.7776) (-38.5146, 37.7687) knots 0 0 0 0 1 1 1 1
  line L501 (-38.5146, 37.7687) -> (-38.5146, 41.417)
  spline S819 degree 3 poles (-39.4568, 41.0806) (-39.4944, 41.0656) (-39.532, 41.0538) (-39.5696, 41.0366) knots 0 0 0 0 1 1 1 1
  line L502 (-39.5696, 41.0366) -> (-39.5696, 37.6097)
  spline S820 degree 3 poles (-39.5696, 37.6097) (-39.5309, 37.6247) (-39.4933, 37.6366) (-39.4568, 37.6494) knots 0 0 0 0 1 1 1 1
  line L503 (-39.4568, 37.6494) -> (-39.4568, 41.0806)
  line L504 (-38.8283, 41.3117) -> (-38.9411, 41.2741)
  line L505 (-38.9411, 41.2741) -> (-38.9411, 37.7795)
  spline S821 degree 3 poles (-38.9411, 37.7795) (-38.8971, 37.7859) (-38.8606, 37.7902) (-38.8283, 37.7924) knots 0 0 0 0 1 1 1 1
  line L506 (-38.8283, 37.7924) -> (-38.8283, 41.3117)
  spline S822 degree 3 poles (-39.1431, 41.201) (-39.1806, 41.1877) (-39.2179, 41.1738) (-39.2548, 41.1592) knots 0 0 0 0 1 1 1 1
  line L507 (-39.2548, 41.1592) -> (-39.2548, 37.7108)
  spline S823 degree 3 poles (-39.2548, 37.7108) (-39.2162, 37.7215) (-39.1786, 37.7321) (-39.1431, 37.7398) knots 0 0 0 0 1 1 1 1
  line L508 (-39.1431, 37.7398) -> (-39.1431, 41.201)
  spline S824 degree 3 poles (-39.7716, 40.9549) (-39.8081, 40.9377) (-39.8457, 40.9237) (-39.8833, 40.9087) knots 0 0 0 0 1 1 1 1
  line L509 (-39.8833, 40.9087) -> (-39.8833, 37.4829)
  line L510 (-39.8833, 37.4829) -> (-39.7716, 37.5312)
  line L511 (-39.7716, 37.5312) -> (-39.7716, 40.9549)
  spline S825 degree 3 poles (-37.2577, 41.763) (-37.2953, 41.7544) (-37.3329, 41.7436) (-37.3694, 41.7361) knots 0 0 0 0 1 1 1 1
  line L512 (-37.3694, 41.7361) -> (-37.3694, 37.0949)
  line L513 (-37.3694, 37.0949) -> (-37.2577, 37.1261)
  line L514 (-37.2577, 37.1261) -> (-37.2577, 41.763)
  line L515 (-34.429, 42.1768) -> (-34.5429, 42.1702)
  line L516 (-34.5429, 42.1702) -> (-34.5429, 37.715)
  spline S826 degree 3 poles (-34.5429, 37.715) (-34.5021, 37.7236) (-34.4645, 37.7321) (-34.429, 37.7365) knots 0 0 0 0 1 1 1 1
  line L517 (-34.429, 37.7365) -> (-34.429, 42.1768)
  spline S827 degree 3 poles (-35.0575, 42.1262) (-35.0951, 42.124) (-35.1327, 42.1176) (-35.1692, 42.1134) knots 0 0 0 0 1 1 1 1
  line L518 (-35.1692, 42.1134) -> (-35.1692, 37.4647)
  spline S828 degree 3 poles (-35.1692, 37.4647) (-35.1306, 37.4818) (-35.093, 37.5001) (-35.0575, 37.5195) knots 0 0 0 0 1 1 1 1
  line L519 (-35.0575, 37.5195) -> (-35.0575, 42.1262)
  line L520 (-34.7438, 42.153) -> (-34.8555, 42.1445)
  line L521 (-34.8555, 42.1445) -> (-34.8555, 37.6064)
  line L522 (-34.8555, 37.6064) -> (-34.7438, 37.6527)
  line L523 (-34.7438, 37.6527) -> (-34.7438, 42.153)
  line L524 (-34.1153, 42.1929) -> (-34.2281, 42.1865)
  line L525 (-34.2281, 42.1865) -> (-34.2281, 37.7182)
  spline S829 degree 3 poles (-34.2281, 37.7182) (-34.1884, 37.7067) (-34.1504, 37.6897) (-34.1153, 37.6677) knots 0 0 0 0 1 1 1 1
  line L526 (-34.1153, 37.6677) -> (-34.1153, 42.1929)
  line L527 (-35.3723, 42.0929) -> (-35.4851, 42.08)
  line L528 (-35.4851, 42.08) -> (-35.4851, 37.3013)
  spline S830 degree 3 poles (-35.4851, 37.3013) (-35.4464, 37.3227) (-35.4088, 37.341) (-35.3723, 37.3604) knots 0 0 0 0 1 1 1 1
  line L529 (-35.3723, 37.3604) -> (-35.3723, 42.0929)
  line L530 (-36.0008, 42.0069) -> (-36.1125, 41.9897)
  line L531 (-36.1125, 41.9897) -> (-36.1125, 36.9692)
  line L532 (-36.1125, 36.9692) -> (-36.0008, 37.0262)
  line L533 (-36.0008, 37.0262) -> (-36.0008, 42.0069)
  line L534 (-30.3445, 24.4717) -> (-30.4573, 24.4738)
  line L535 (-30.4573, 24.4738) -> (-30.4573, 23.3068)
  line L536 (-30.4573, 23.3068) -> (-30.3445, 23.3111)
  line L537 (-30.3445, 23.3111) -> (-30.3445, 24.4717)
  line L538 (-31.2877, 24.4588) -> (-31.3996, 24.4513)
  line L539 (-31.3996, 24.4513) -> (-31.3996, 23.367)
  line L540 (-31.3996, 23.367) -> (-31.2877, 23.353)
  line L541 (-31.2877, 23.353) -> (-31.2877, 24.4588)
  line L542 (-30.9719, 24.4728) -> (-31.0848, 24.4695)
  line L543 (-31.0848, 24.4695) -> (-31.0848, 23.3315)
  line L544 (-31.0848, 23.3315) -> (-30.9719, 23.3208)
  line L545 (-30.9719, 23.3208) -> (-30.9719, 24.4728)
  line L546 (-29.0887, 24.4147) -> (-29.2003, 24.4201)
  line L547 (-29.2003, 24.4201) -> (-29.2003, 23.252)
  spline S831 degree 3 poles (-29.2003, 23.252) (-29.1638, 23.2499) (-29.1263, 23.2445) (-29.0887, 23.2402) knots 0 0 0 0 1 1 1 1
  line L548 (-29.0887, 23.2402) -> (-29.0887, 24.4147)
  line L549 (-29.4024, 24.4309) -> (-29.426, 24.4319)
  line L550 (-29.426, 24.4319) -> (-29.5151, 24.4362)
  line L551 (-29.5151, 24.4362) -> (-29.5151, 23.2821)
  line L552 (-29.5151, 23.2821) -> (-29.4024, 23.2724)
  line L553 (-29.4024, 23.2724) -> (-29.4024, 24.4309)
  line L554 (-30.0309, 24.462) -> (-30.1436, 24.4663)
  line L555 (-30.1436, 24.4663) -> (-30.1436, 23.3133)
  line L556 (-30.1436, 23.3133) -> (-30.0309, 23.3111)
  line L557 (-30.0309, 23.3111) -> (-30.0309, 24.462)
  line L558 (-29.7172, 24.447) -> (-29.8288, 24.4524)
  line L559 (-29.8288, 24.4524) -> (-29.8288, 23.3025)
  line L560 (-29.8288, 23.3025) -> (-29.7172, 23.2961)
  line L561 (-29.7172, 23.2961) -> (-29.7172, 24.447)
  line L562 (-30.6582, 24.476) -> (-30.7711, 24.476)
  line L563 (-30.7711, 24.476) -> (-30.7711, 23.3068)
  line L564 (-30.7711, 23.3068) -> (-30.6582, 23.3025)
  line L565 (-30.6582, 23.3025) -> (-30.6582, 24.476)
  line L566 (-31.6004, 24.4341) -> (-31.7133, 24.4201)
  line L567 (-31.7133, 24.4201) -> (-31.7133, 23.41)
  line L568 (-31.7133, 23.41) -> (-31.6004, 23.3939)
  line L569 (-31.6004, 23.3939) -> (-31.6004, 24.4341)
  line L570 (-33.1721, 24.0064) -> (-33.2849, 23.9441)
  line L571 (-33.2849, 23.9441) -> (-33.2849, 23.6776)
  line L572 (-33.2849, 23.6776) -> (-33.1721, 23.6561)
  line L573 (-33.1721, 23.6561) -> (-33.1721, 24.0064)
  line L574 (-33.4869, 23.8162) -> (-33.5986, 23.7399)
  spline S832 degree 3 poles (-33.5986, 23.7399) (-33.5612, 23.7332) (-33.5239, 23.7246) (-33.4869, 23.7163) knots 0 0 0 0 1 1 1 1
  line L575 (-33.4869, 23.7163) -> (-33.4869, 23.8162)
  spline S833 degree 3 poles (-32.8574, 24.1493) (-32.8951, 24.1342) (-32.9328, 24.1184) (-32.9701, 24.102) knots 0 0 0 0 1 1 1 1
  line L576 (-32.9701, 24.102) -> (-32.9701, 23.6185)
  line L577 (-32.9701, 23.6185) -> (-32.8574, 23.5991)
  line L578 (-32.8574, 23.5991) -> (-32.8574, 24.1493)
  line L579 (-32.5437, 24.2568) -> (-32.6564, 24.2213)
  line L580 (-32.6564, 24.2213) -> (-32.6564, 23.5626)
  line L581 (-32.6564, 23.5626) -> (-32.5437, 23.5433)
  line L582 (-32.5437, 23.5433) -> (-32.5437, 24.2568)
  line L583 (-31.9152, 24.3943) -> (-32.0279, 24.375)
  line L584 (-32.0279, 24.375) -> (-32.0279, 23.4573)
  line L585 (-32.0279, 23.4573) -> (-31.9152, 23.4401)
  line L586 (-31.9152, 23.4401) -> (-31.9152, 24.3943)
  line L587 (-32.23, 24.3363) -> (-32.3416, 24.3105)
  line L588 (-32.3416, 24.3105) -> (-32.3416, 23.5089)
  line L589 (-32.3416, 23.5089) -> (-32.23, 23.4895)
  line L590 (-32.23, 23.4895) -> (-32.23, 24.3363)
  spline S834 degree 3 poles (-26.5749, 26.6972) (-26.6112, 26.7101) (-26.6489, 26.7219) (-26.6865, 26.7326) knots 0 0 0 0 1 1 1 1
  line L591 (-26.6865, 26.7326) -> (-26.6865, 22.4934)
  spline S835 degree 3 poles (-26.6865, 22.4934) (-26.6489, 22.4677) (-26.6117, 22.4415) (-26.5749, 22.4149) knots 0 0 0 0 1 1 1 1
  line L592 (-26.5749, 22.4149) -> (-26.5749, 26.6972)
  spline S836 degree 3 poles (-25.9464, 25.83) (-25.987, 25.862) (-26.0247, 25.8976) (-26.0591, 25.9364) knots 0 0 0 0 1 1 1 1
  line L593 (-26.0591, 25.9364) -> (-26.0591, 22.0399)
  line L594 (-26.0591, 22.0399) -> (-25.9464, 21.9561)
  line L595 (-25.9464, 21.9561) -> (-25.9464, 25.83)
  spline S837 degree 3 poles (-25.6316, 25.7472) (-25.6686, 25.7387) (-25.7067, 25.7368) (-25.7443, 25.7419) knots 0 0 0 0 1 1 1 1
  line L596 (-25.7443, 25.7419) -> (-25.7443, 21.8056)
  line L597 (-25.7443, 21.8056) -> (-25.6316, 21.7229)
  line L598 (-25.6316, 21.7229) -> (-25.6316, 25.7472)
  spline S838 degree 3 poles (-26.2601, 26.2416) (-26.2922, 26.306) (-26.3158, 26.3576) (-26.3266, 26.3834) knots 0 0 0 0 1 1 1 1
  spline S839 degree 3 poles (-26.3266, 26.3834) (-26.3366, 26.4073) (-26.3383, 26.4338) (-26.3317, 26.4589) knots 0 0 0 0 1 1 1 1
  spline S840 degree 3 poles (-26.3317, 26.4589) (-26.3252, 26.4839) (-26.3105, 26.5061) (-26.29, 26.522) knots 0 0 0 0 1 1 1 1
  spline S841 degree 3 poles (-26.29, 26.522) (-26.2815, 26.5285) (-26.2697, 26.5338) (-26.2612, 26.5381) knots 0 0 0 0 1 1 1 1
  line L599 (-26.2612, 26.5381) -> (-26.2612, 26.5629)
  spline S842 degree 3 poles (-26.2612, 26.5629) (-26.2978, 26.5832) (-26.3355, 26.6018) (-26.3739, 26.6187) knots 0 0 0 0 1 1 1 1
  line L600 (-26.3739, 26.6187) -> (-26.3739, 22.2709)
  spline S843 degree 3 poles (-26.3739, 22.2709) (-26.3363, 22.2451) (-26.2986, 22.2161) (-26.2612, 22.1893) knots 0 0 0 0 1 1 1 1
  line L601 (-26.2612, 22.1893) -> (-26.2601, 26.2416)
  spline S844 degree 3 poles (-24.6894, 24.317) (-24.7259, 24.3892) (-24.7635, 24.4608) (-24.8023, 24.5319) knots 0 0 0 0 1 1 1 1
  line L602 (-24.8023, 24.5319) -> (-24.8023, 21.1319)
  spline S845 degree 3 poles (-24.8023, 21.1319) (-24.7649, 21.1076) (-24.7273, 21.084) (-24.6894, 21.0609) knots 0 0 0 0 1 1 1 1
  line L603 (-24.6894, 21.0609) -> (-24.6894, 24.317)
  spline S846 degree 3 poles (-24.4875, 20.9546) (-24.4825, 20.9534) (-24.4778, 20.9516) (-24.4734, 20.9492) knots 0 0 0 0 1 1 1 1
  line L604 (-24.4734, 20.9492) -> (-24.2521, 21.0985)
  line L605 (-24.2521, 21.0985) -> (-24.2521, 22.9361)
  spline S847 degree 3 poles (-24.2521, 22.9361) (-24.3532, 23.1048) (-24.4283, 23.2907) (-24.4875, 23.4702) knots 0 0 0 0 1 1 1 1
  line L606 (-24.4875, 23.4702) -> (-24.4875, 20.9546)
  line L607 (-25.0031, 24.8908) -> (-25.1158, 25.081)
  line L608 (-25.1158, 25.081) -> (-25.1158, 21.3468)
  line L609 (-25.1158, 21.3468) -> (-25.0031, 21.2683)
  line L610 (-25.0031, 21.2683) -> (-25.0031, 24.8908)
  line L611 (-25.3179, 25.4055) -> (-25.4295, 25.5785)
  line L612 (-25.4295, 25.5785) -> (-25.4295, 21.5735)
  line L613 (-25.4295, 21.5735) -> (-25.3179, 21.4908)
  line L614 (-25.3179, 21.4908) -> (-25.3179, 25.4055)
  spline S848 degree 3 poles (-28.1443, 24.419) (-28.1821, 24.4136) (-28.2202, 24.4093) (-28.2581, 24.4061) knots 0 0 0 0 1 1 1 1
  line L615 (-28.2581, 24.4061) -> (-28.2581, 23.1134)
  spline S849 degree 3 poles (-28.2581, 23.1134) (-28.2196, 23.107) (-28.183, 23.0994) (-28.1443, 23.0908) knots 0 0 0 0 1 1 1 1
  line L616 (-28.1443, 23.0908) -> (-28.1443, 24.419)
  spline S850 degree 3 poles (-27.8317, 24.4943) (-27.8682, 24.4824) (-27.9048, 24.4706) (-27.9435, 24.4599) knots 0 0 0 0 1 1 1 1
  line L617 (-27.9435, 24.4599) -> (-27.9435, 23.0468)
  line L618 (-27.9435, 23.0468) -> (-27.8317, 23.0188)
  line L619 (-27.8317, 23.0188) -> (-27.8317, 24.4943)
  spline S851 degree 3 poles (-26.8884, 25.5033) (-26.9193, 25.41) (-26.957, 25.3192) (-27.0013, 25.2314) knots 0 0 0 0 1 1 1 1
  line L620 (-27.0013, 25.2314) -> (-27.0013, 22.6997)
  spline S852 degree 3 poles (-27.0013, 22.6997) (-26.9648, 22.6782) (-26.9282, 22.6546) (-26.8884, 22.6288) knots 0 0 0 0 1 1 1 1
  line L621 (-26.8884, 22.6288) -> (-26.8884, 25.5033)
  line L622 (-28.4591, 24.3965) -> (-28.4655, 24.3965)
  line L623 (-28.4655, 24.3965) -> (-28.574, 24.3975)
  line L624 (-28.574, 24.3975) -> (-28.574, 23.1693)
  line L625 (-28.574, 23.1693) -> (-28.4602, 23.1499)
  line L626 (-28.4602, 23.1499) -> (-28.4602, 24.3965)
  line L627 (-28.4602, 24.3965) -> (-28.4591, 24.3965)
  line L628 (-28.7739, 24.4019) -> (-28.8866, 24.4061)
  line L629 (-28.8866, 24.4061) -> (-28.8866, 23.2155)
  line L630 (-28.8866, 23.2155) -> (-28.7739, 23.1994)
  line L631 (-28.7739, 23.1994) -> (-28.7739, 24.4019)
  spline S853 degree 3 poles (-27.2032, 24.923) (-27.238, 24.881) (-27.2753, 24.8411) (-27.315, 24.8038) knots 0 0 0 0 1 1 1 1
  line L632 (-27.315, 24.8038) -> (-27.315, 22.8566)
  line L633 (-27.315, 22.8566) -> (-27.2032, 22.8082)
  line L634 (-27.2032, 22.8082) -> (-27.2032, 24.923)
  spline S854 degree 3 poles (-27.5169, 24.6458) (-27.5536, 24.6223) (-27.5912, 24.6004) (-27.6298, 24.5802) knots 0 0 0 0 1 1 1 1
  line L635 (-27.6298, 24.5802) -> (-27.6298, 22.964)
  spline S855 degree 3 poles (-27.6298, 22.964) (-27.592, 22.9525) (-27.5544, 22.9407) (-27.5169, 22.9286) knots 0 0 0 0 1 1 1 1
  line L636 (-27.5169, 22.9286) -> (-27.5169, 24.6458)
  spline S856 degree 3 poles (-27.4997, 25.0455) (-27.0367, 25.5087) (-27.0389, 26.3415) (-27.0389, 26.6983) knots 0 0 0 0 1 1 1 1
  line L637 (-27.0389, 26.6983) -> (-27.0389, 26.81)
  line L638 (-27.0389, 26.81) -> (-27.1055, 26.8197)
  line L639 (-27.1055, 26.8197) -> (-27.1055, 26.7982)
  spline S857 degree 3 poles (-27.1055, 26.7982) (-27.1055, 26.3469) (-27.1678, 25.527) (-27.59, 25.1057) knots 0 0 0 0 1 1 1 1
  spline S858 degree 3 poles (-27.59, 25.1057) (-27.6777, 25.0166) (-27.7827, 24.9464) (-27.8985, 24.8995) knots 0 0 0 0 1 1 1 1
  spline S859 degree 3 poles (-27.8985, 24.8995) (-28.0144, 24.8525) (-28.1387, 24.8298) (-28.2636, 24.8328) knots 0 0 0 0 1 1 1 1
  spline S860 degree 3 poles (-28.2636, 24.8328) (-28.7213, 24.8328) (-29.1724, 25.0681) (-29.743, 25.3647) knots 0 0 0 0 1 1 1 1
  spline S861 degree 3 poles (-29.743, 25.3647) (-30.3972, 25.7053) (-31.2136, 26.1298) (-32.3482, 26.3469) knots 0 0 0 0 1 1 1 1
  spline S862 degree 3 poles (-32.3482, 26.3469) (-33.1259, 26.4941) (-35.1327, 26.5811) (-35.7633, 26.6058) knots 0 0 0 0 1 1 1 1
  line L640 (-35.7633, 26.6058) -> (-35.5066, 26.3329)
  spline S863 degree 2 poles (-35.5066, 26.3329) (-35.3669, 26.4361) (-35.2971, 26.2265) knots 0 0 0 1 1 1
  spline S864 degree 2 poles (-35.2971, 26.2265) (-35.2799, 26.3608) (-35.0618, 26.1094) knots 0 0 0 1 1 1
  spline S865 degree 2 poles (-35.0618, 26.1094) (-34.9103, 26.3275) (-34.8609, 26.0256) knots 0 0 0 1 1 1
  spline S866 degree 2 poles (-34.8609, 26.0256) (-34.7094, 26.1932) (-34.6256, 25.8579) knots 0 0 0 1 1 1
  spline S867 degree 2 poles (-34.6256, 25.8579) (-34.2389, 26.4447) (-34.3732, 25.7902) knots 0 0 0 1 1 1
  spline S868 degree 2 poles (-34.3732, 25.7902) (-34.038, 26.2609) (-34.1551, 25.7225) knots 0 0 0 1 1 1
  spline S869 degree 2 poles (-34.1551, 25.7225) (-33.937, 26.0761) (-33.8704, 25.6226) knots 0 0 0 1 1 1
  spline S870 degree 2 poles (-33.8704, 25.6226) (-33.5352, 26.2942) (-33.6179, 25.5893) knots 0 0 0 1 1 1
  spline S871 degree 2 poles (-33.6179, 25.5893) (-33.1657, 26.2609) (-33.3494, 25.4883) knots 0 0 0 1 1 1
  spline S872 degree 2 poles (-33.3494, 25.4883) (-32.8122, 26.5285) (-33.0636, 25.4044) knots 0 0 0 1 1 1
  spline S873 degree 2 poles (-33.0636, 25.4044) (-32.5597, 26.479) (-32.7779, 25.2701) knots 0 0 0 1 1 1
  spline S874 degree 2 poles (-32.7779, 25.2701) (-32.0558, 26.5467) (-32.5426, 25.1014) knots 0 0 0 1 1 1
  spline S875 degree 2 poles (-32.5426, 25.1014) (-31.5993, 26.4866) (-32.173, 25.2024) knots 0 0 0 1 1 1
  spline S876 degree 2 poles (-32.173, 25.2024) (-31.3501, 26.1599) (-31.8035, 25.3034) knots 0 0 0 1 1 1
  spline S877 degree 2 poles (-31.8035, 25.3034) (-30.9644, 26.0084) (-31.6519, 25.0348) knots 0 0 0 1 1 1
  spline S878 degree 2 poles (-31.6519, 25.0348) (-30.6947, 25.9922) (-31.2158, 25.1014) knots 0 0 0 1 1 1
  spline S879 degree 2 poles (-31.2158, 25.1014) (-30.3455, 25.8579) (-30.9676, 24.9843) knots 0 0 0 1 1 1
  spline S880 degree 2 poles (-30.9676, 24.9843) (-30.2629, 25.6892) (-30.5315, 25.0681) knots 0 0 0 1 1 1
  spline S881 degree 2 poles (-30.5315, 25.0681) (-30.0276, 25.3196) (-30.1963, 24.9338) knots 0 0 0 1 1 1
  spline S882 degree 2 poles (-30.1963, 24.9338) (-29.7762, 25.269) (-29.8095, 24.8671) knots 0 0 0 1 1 1
  spline S883 degree 2 poles (-29.8095, 24.8671) (-29.3573, 25.2207) (-29.4744, 24.7661) knots 0 0 0 1 1 1
  spline S884 degree 3 poles (-29.4744, 24.7661) (-29.1209, 24.9359) (-29.0843, 24.7898) (-29.0843, 24.7167) knots 0 0 0 0 1 1 1 1
  spline S885 degree 3 poles (-29.0843, 24.7167) (-28.8642, 24.707) (-28.6568, 24.6984) (-28.4666, 24.6984) knots 0 0 0 0 1 1 1 1
  spline S886 degree 3 poles (-28.4666, 24.6984) (-28.0552, 24.6995) (-27.7297, 24.8156) (-27.4997, 25.0455) knots 0 0 0 0 1 1 1 1
  spline S887 degree 3 poles (-27.4986, 39.2635) (-27.5111, 39.2488) (-27.5275, 39.2381) (-27.5459, 39.2323) knots 0 0 0 0 1 1 1 1
  spline S888 degree 3 poles (-27.5459, 39.2323) (-27.5567, 39.2302) (-27.7984, 39.1442) (-27.7984, 38.7746) knots 0 0 0 0 1 1 1 1